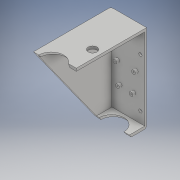
# Autodesk Inventor part: Center_bar_panel
Saved by Autodesk Inventor 2019 (Build 230136000, 136)
## iProperties
Created: 2019-11-07
Part Number: Center_bar_panel
Material: Generic
Document SubType Name: Modeling
Designer: steve
Density: 1 g/cm^3
Appearance: Default
Author: steve
Autodesk Inventor part; units mm, degrees
ref_plane "YZ Plane" through (0, 0, 0) normal (1, 0, 0) x (0, 1, 0)
ref_plane "XY Plane" through (0, 0, 0) normal (0, 0, 1) x (1, 0, 0)
sketch "Sketch1" plane through (0, 0, 0) normal (0, 1, 0) x (-1, 0, 0)
  arc A0 (-22.75, 0) -> (22.75, 0) centre (0, 0) ccw
  line L0 (32.75, 0) -> (32.75, -28)
  line L1 (32.75, -28) -> (-32.75, -28)
  line L2 (-32.75, -28) -> (-32.75, 0)
  line L3 (-32.75, 0) -> (-22.75, 0)
  line L4 (22.75, 0) -> (32.75, 0)
  line L5 (45.85, 0) -> (-45.85, 0) projected
  dimension "d1" = 10
  dimension "archRad" = 22.75
  dimension "d3" = 28
  dimension "d71" = 65.5
  dimension "d72" = 55.5
  constraints: 10 end point, 3 perpendicular, 2 collinear, 2 equal length, 2 point on circle, 1 centre point, 1 coincident, 1 vertical
  measures "d1" distance of L4.start L0.start
  measures "archRad" radius of A0
  measures "d3" distance from line of A0.centre L1
  measures "d71" distance of L0.end L1.end
  measures "d72" distance of L2.end L4.start
ref_plane "Work Plane1" through (0, 5, 0) normal (0, 1, 0) x (-1, 0, 0)
sketch "Sketch2" plane through (0, 5, 0) normal (0, 1, 0) x (-1, 0, 0)
  line L0 (32.75, -28) -> (-32.75, -28) projected
  line L1 (32.75, 0) -> (32.75, -28) projected
  line L2 (-32.75, -28) -> (-32.75, 0) projected
  line L3 (32.75, 0) -> (32.75, 3.575)
  line L4 (-32.75, 3.575) -> (-32.75, 0)
  arc A0 (-22.75, 3.575) -> (22.75, 3.575) centre (0, 3.575) ccw
  line L5 (32.75, 3.575) -> (22.75, 3.575)
  line L6 (-22.75, 3.575) -> (-32.75, 3.575)
  line L7 (22.75, 3.575) -> (-22.75, 3.575) construction
  point P0 (0, 0)
  dimension "d5" = 22.75
  dimension "d6" = 3.575
  constraints: 10 end point, 2 collinear, 2 horizontal, 2 point on circle, 2 vertical, 1 centre point, 1 coincident, 1 midpoint
  measures "d5" radius of A0
  measures "d6" distance from line of L5 L1.start
loft "Loft1" add profiles "Sketch1", "Sketch2" contours A0 L4 L0 L1 L2 L3 / all
sketch "Sketch3" plane through (0, 5, 3.575) normal (0, 1, 0) x (1, 0, 0)
  line L0 (32.75, 31.575) -> (32.75, 3.575) projected
  line L1 (-32.75, 31.575) -> (32.75, 31.575)
  line L2 (32.75, 31.575) -> (32.75, 28.325)
  line L3 (32.75, 28.325) -> (-32.75, 28.325)
  line L4 (-32.75, 28.325) -> (-32.75, 31.575)
  point P0 (0, 3.575)
  dimension "d12" = 3.25
  constraints: 8 end point, 2 parallel, 1 horizontal, 1 perpendicular, 1 point on line
  measures "d12" distance between parallel lines of L1 L3
extrude "Extrusion1" add sketch "Sketch3" along normal blind 150
sketch "Sketch4" plane through (-32.75, 5, -24.75) normal (0, 0, 1) x (1, 0, 0)
  line L0 (45.25, 43.2269) -> (20.25, 43.2269) construction
  line L1 (15.75, 80.2269) -> (49.75, 80.2269) construction
  line L2 (55.5, -5) -> (10, -5) construction
  line L3 (65.5, 0) -> (65.5, 150) construction
  line L4 (0, 0) -> (0, 150) construction
  circle A0 centre (20.25, 43.2269) radius 3.5
  circle A1 centre (45.25, 43.2269) radius 3.5
  circle A2 centre (49.75, 80.2269) radius 3.5
  circle A3 centre (15.75, 80.2269) radius 3.5
  circle A4 centre (20.25, 43.2269) radius 1
  circle A5 centre (45.25, 43.2269) radius 1
  circle A6 centre (49.75, 80.2269) radius 1
  circle A7 centre (15.75, 80.2269) radius 1
  point P0 (32.75, -5)
  dimension "d15" = 25
  dimension "d18" = 65.5
  dimension "d20" = 2.5
  dimension "d21" = 2
  dimension "d65" = 34
  dimension "d66" = 15.75
  dimension "d67" = 20.25
  dimension "d124" = 37
  constraints: 8 centre point, 7 coincident, 6 equal radius, 4 end point, 1 concentric, 1 horizontal, 1 parallel
  measures "d15" distance of L0.start L0.end
  measures "d18" distance between parallel lines of L3 L4
  measures "d20" radial gap between concentric circles of A4 A0
  measures "d21" diameter of A4
  measures "d65" distance of L1.start L1.end
  measures "d66" distance from line of L4 L1.start
  measures "d67" distance from line of L4 L0.end
  measures "d124" vertical distance of L0.start L1.end
extrude "Extrusion2" add sketch "Sketch4" along normal blind 5
sketch "Sketch5" plane through (32.75, 0, -28) normal (0, 0, -1) x (-1, 0, 0)
  line L0 (49.75, 51.2269) -> (15.75, 51.2269)
  line L1 (15.75, 51.2269) -> (15.75, 88.2269)
  line L2 (15.75, 88.2269) -> (49.75, 88.2269)
  line L3 (49.75, 88.2269) -> (49.75, 51.2269)
  line L4 (49.75, 51.2269) -> (15.75, 88.2269) construction
  line L5 (15.75, 51.2269) -> (49.75, 88.2269) construction
  circle A0 centre (45.25, 48.2269) radius 3.5 projected
  circle A1 centre (20.25, 48.2269) radius 3.5 projected
  line L6 (65.5, 0) -> (0, 0) projected
  line L7 (65.5, 0) -> (65.5, 155) projected
  line L8 (0, 155) -> (65.5, 155) projected
  line L9 (0, 0) -> (0, 155) projected
  circle A2 centre (15.75, 85.2269) radius 3.5 projected
  circle A3 centre (49.75, 85.2269) radius 3.5 projected
  line L10 (13.75, 49.2269) -> (51.75, 49.2269)
  line L11 (51.75, 49.2269) -> (51.75, 90.2269)
  line L12 (51.75, 90.2269) -> (13.75, 90.2269)
  line L13 (13.75, 90.2269) -> (13.75, 49.2269)
  point P0 (32.75, 0)
  point P1 (32.75, 69.7269)
  dimension "d125" = 2
  constraints: 20 end point, 4 parallel, 3 vertical alignment, 2 midpoint, 2 perpendicular, 1 horizontal, 6 other
  measures "d125" distance between parallel lines of L13 L1
sketch "Sketch6" plane through (0, 155, 3.575) normal (0, 1, 0) x (1, 0, 0)
  line L0 (32.75, 31.575) -> (-32.75, 31.575) projected
  line L1 (-32.75, 31.575) -> (-32.75, -107.25)
  line L2 (32.75, 28.325) -> (32.75, 31.575) projected
  line L3 (32.75, 31.575) -> (32.75, -107.25)
  arc A0 (22.75, -107.25) -> (-22.75, -107.25) centre (0, -107.25) ccw
  line L4 (-32.75, -107.25) -> (-22.75, -107.25)
  line L5 (22.75, -107.25) -> (32.75, -107.25)
  line L6 (-22.75, 0) -> (-32.75, 0) projected
  line L7 (32.75, 0) -> (22.75, 0) projected
  point P0 (0, 3.575)
  dimension "d27" = 22.75
  dimension "d28" = 107.25
  constraints: 8 end point, 2 collinear, 2 equal length, 2 point on circle, 2 vertical, 1 centre point, 1 horizontal
  measures "d27" radius of A0
  measures "d28" distance between parallel lines of L7 L5
ref_plane "Work Plane3" through (0, 160, 3.575) normal (0, 1, 0) x (1, 0, 0)
sketch "Sketch7" plane through (0, 160, 3.575) normal (0, 1, 0) x (1, 0, 0)
  line L0 (32.75, 31.575) -> (-32.75, 31.575) projected
  line L1 (-32.75, 31.575) -> (-32.75, -107.25) projected
  line L2 (32.75, 31.575) -> (32.75, -107.25) projected
  line L3 (-32.75, -107.25) -> (-32.75, -110.825)
  arc A0 (22.75, -110.825) -> (-22.75, -110.825) centre (0, -110.825) ccw
  line L4 (-32.75, -110.825) -> (-22.75, -110.825)
  line L5 (22.75, -110.825) -> (32.75, -110.825)
  line L6 (32.75, -110.825) -> (32.75, -107.25)
  line L7 (-22.75, -110.825) -> (22.75, -110.825) construction
  point P0 (0, 3.575)
  point P1 (50, -9)
  dimension "d37" = 3.575
  dimension "d38" = 22.75
  constraints: 10 end point, 2 equal length, 2 point on circle, 1 centre point, 1 coincident, 1 collinear, 1 horizontal, 1 midpoint, 1 perpendicular, 1 point on line, 1 vertical
  measures "d37" distance of L1.end L3.end
  measures "d38" radius of A0
loft "Loft2" add profiles "Sketch6", "Sketch7"
sketch "Sketch8" plane through (0, 160, 114.4) normal (0, 1, 0) x (1, 0, 0)
  circle A0 centre (18, 58) radius 8
  point P0 (0, 114.4)
  dimension "d116" = 16
  constraints: 1 centre point
  measures "d116" diameter of A0
extrude "Extrusion4" cut sketch "Sketch8" against normal up to next
sketch "Sketch9" plane through (-32.75, 0, -28) normal (-1, 0, 0) x (0, 0, 1)
  line L0 (31.575, 5) -> (3.25, 5) projected
  line L1 (3.25, 155) -> (138.825, 155) projected
  line L2 (3.25, 5) -> (3.25, 155) projected
  line L3 (138.825, 155) -> (142.4, 160) projected
  line L4 (31.575, 5) -> (138.825, 155)
  point P0 (28, 0)
  constraints: 2 end point, 1 collinear
extrude "Extrusion5" add sketch "Sketch9" against normal blind 5
sketch "Sketch10" plane through (32.75, 5, -24.75) normal (0, 0, 1) x (1, 0, 0)
  line L0 (-11, 136) -> (-5, 136)
  line L1 (-5, 136) -> (-5, 118)
  line L2 (-5, 118) -> (-11, 118)
  line L3 (-11, 118) -> (-11, 136)
  line L4 (-11, 38) -> (-5, 38)
  line L5 (-5, 38) -> (-5, 20)
  line L6 (-5, 20) -> (-11, 20)
  line L7 (-11, 20) -> (-11, 38)
  line L8 (0, 0) -> (0, 150) projected
  line L9 (0, 0) -> (-10, 0) projected
  point P0 (-32.75, -5)
  dimension "d47" = 80
  dimension "d48" = 6
  dimension "d49" = 18
  dimension "d50" = 5
  dimension "d51" = 20
  constraints: 16 end point, 4 parallel, 2 horizontal, 2 perpendicular, 2 point on line, 1 collinear
  measures "d47" distance between parallel lines of L4 L2
  measures "d48" distance of L0.start L0.end
  measures "d49" distance of L0.end L1.end
  measures "d50" distance between parallel lines of L8 L1
  measures "d51" distance between parallel lines of L9 L6
extrude "Extrusion6" [suppressed]
sketch "Sketch11" plane through (27.75, 190, -65) normal (1, 0, 0) x (0, 0, -1)
  circle A0 centre (-62.625, -55) radius 4
  circle A1 centre (-62.625, -153) radius 4
  line L0 (-47, -162) -> (-72, -162) projected
  line L1 (-47, -144) -> (-72, -144) projected
  line L2 (-47, -182) -> (-47, -32) projected
  line L3 (-72, -162) -> (-72, -144) projected
  line L4 (-47, -64) -> (-72, -64) projected
  line L5 (-47, -46) -> (-72, -46) projected
  point P0 (-65, -190)
  dimension "d54" = 18
  dimension "d55" = 25
  dimension "d56" = 9.375
  dimension "d57" = 9
  dimension "d58" = 0
  dimension "d59" = 18
  dimension "d60" = 9
  dimension "d61" = 8
  constraints: 2 centre point, 1 equal radius
  measures "d54" distance between parallel lines of L0 L1
  measures "d55" distance between parallel lines of L2 L3
  measures "d56" distance from line of L3 A1.centre
  measures "d57" distance from line of A1.centre L1
  measures "d58" horizontal distance of A1.centre A0.centre
  measures "d59" distance between parallel lines of L4 L5
  measures "d60" distance from line of L5 A0.centre
  measures "d61" diameter of A1
extrude "Extrusion7" [suppressed]
fillet "Fillet1" [suppressed]
fillet "Fillet2" radius 4.5 1 edges at (-32.75, 0, -14)
fillet "Fillet3" radius 4.5 3 edges at (-31.432, 1.318, -28) (2.25, 0, -28) (-32.75, 82.25, -28)
sketch "Sketch12" plane through (-32.75, 4.5, -23.5) normal (-1, 0, 0) x (0, 0, 1)
  line L0 (60.5939, 215.8444) -> (62.2991, 204.7949) construction
  line L1 (62.2991, 204.7949) -> (81.807, 216.246) construction
  line L2 (41.3847, 184.2911) -> (56.7371, 199.246) construction
  line L3 (56.7371, 199.246) -> (61.2816, 185.5477) construction
  line L4 (61.2816, 185.5477) -> (81.807, 216.246) construction
  line L5 (41.3847, 184.2911) -> (37.3847, 196.2911) construction
  line L6 (37.3847, 196.2911) -> (18.3847, 178.9195) construction
  line L7 (18.3847, 178.9195) -> (18.3847, 201.9388) construction
  line L8 (18.3847, 201.9388) -> (43.3847, 219.7249) construction
  line L9 (43.3847, 219.7249) -> (45.3847, 201.9388) construction
  line L10 (45.3847, 201.9388) -> (60.5939, 215.8444) construction
  line L11 (21.9472, 62.1913) -> (9.1489, 77.7659)
  line L12 (9.1489, 77.7659) -> (34.9472, 116.1822)
  line L13 (34.9472, 116.1822) -> (41.2994, 100.2139)
  line L14 (52.9194, 125.0534) -> (63.4758, 112.4149)
  line L15 (63.4758, 112.4149) -> (86.8697, 137.6919)
  line L16 (55.8147, 101.6972) -> (63.9472, 87.138)
  line L17 (63.9472, 87.138) -> (86.8697, 137.6919)
  line L18 (55.8147, 101.6972) -> (40.4622, 68.6972)
  line L19 (40.4622, 68.6972) -> (34.0889, 86.8345)
  line L20 (34.0889, 86.8345) -> (21.9472, 62.1913)
  line L21 (41.2994, 100.2139) -> (52.9194, 125.0534)
  point P0 (23.5, -4.5)
  constraints: 44 end point, 1 parallel, 1 point on line, 1 vertical
extrude "Extrusion8" cut sketch "Sketch12" against normal blind 1
sketch "Sketch13" plane through (32.75, 160, -28) normal (0, 0, -1) x (-1, 0, 0)
  circle A0 centre (8, -135) radius 3
  circle A1 centre (8, -45) radius 3
  line L0 (0, -160) -> (61, -160) projected
  line L1 (0, -155.5) -> (0, 0) projected
  point P0 (32.75, -160)
  dimension "d117" = 25
  dimension "d118" = 8
  dimension "d119" = 8
  dimension "d120" = 45
  dimension "d121" = 6
  constraints: 2 centre point, 1 equal radius
  measures "d117" distance from line of A0.centre L0
  measures "d118" distance from line of L1 A0.centre
  measures "d119" distance from line of L1 A1.centre
  measures "d120" vertical distance of A1.centre L1.end
  measures "d121" diameter of A0
extrude "Extrusion9" cut sketch "Sketch13" against normal up to next
extrude "Extrusion10" cut sketch "Sketch5" against normal blind 0.5 contours L3 A3 L11 L10 A0 L0 | A0 L10 L0 | L3 L2 A3 L11 | A0 L10 A1 L0 | L2 A2 L13 L12 L11 A3 | A1 L10 L0 | L2 L1 A2 L13 | A1 L10 L13 A2 L1 L0
sketch "Sketch14" plane through (0, 160, 114.4) normal (0, 1, 0) x (1, 0, 0)
  arc A0 (22.75, 0) -> (-22.75, 0) centre (0, 0) ccw projected
  line L0 (22.75, 0) -> (32.75, 0) projected
  line L1 (32.75, 0) -> (32.75, 142.4) projected
  line L2 (18.4229, 13.3476) -> (32.75, 13.3513)
  line L3 (32.75, 3.575) -> (32.75, 139.15) projected
  point P0 (0, 114.4)
  constraints: 2 end point, 1 point on circle, 1 point on line
extrude "Extrusion11" cut sketch "Sketch14" against normal up to next
equation "\"d5\" = archRad"
equation "\"d66\" = -0.5 * d65 + 0.5 * d18"
equation "\"d67\" = -0.5 * d15 + 0.5 * d18"
equation "\"d27\" = archRad"
equation "\"d38\" = archRad"
equation "\"d56\" = 0.375 * d55"
equation "\"d57\" = 0.5 * d54"
equation "\"d60\" = 0.5 * d59"
equation "\"archWidth\" = 5"
equation "\"d4\" = archWidth"
equation "\"slope\" = 0.715"
equation "\"d36\" = archWidth"
body "Solid1"
